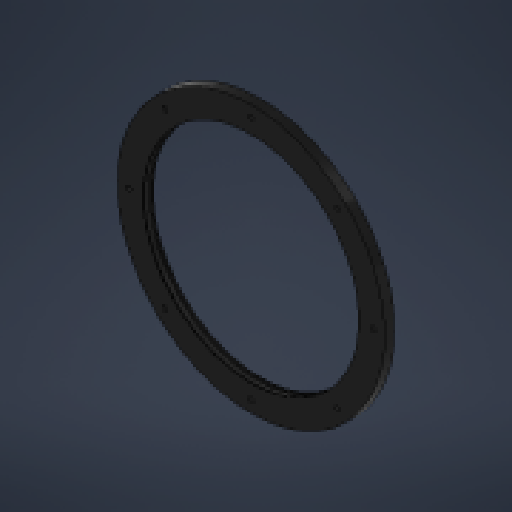
# Autodesk Inventor part: 3DPRINT,TURRET,BEARING,OUTER
Saved by Autodesk Inventor 2026 (Build 300175000, 175)
## iProperties
Created: 2026-02-09
Part Number: 3DPRINT,TURRET,BEARING,OUTER
Material: Nylon 6/6
Document SubType Name: Modeling
Designer: littl
Density: 1.13 g/cm^3
Appearance: Smooth - Black
Mass: 195.023 g
Surface Area: 545.104 cm^2
Volume: 172.587 cm^3
Author: littl
Autodesk Inventor part; units mm, degrees
ref_plane "YZ Plane" through (0, 0, 0) normal (1, 0, 0) x (0, 1, 0)
ref_plane "XZ Plane" through (0, 0, 0) normal (0, 1, 0) x (-1, 0, 0)
ref_plane "XY Plane" through (0, 0, 0) normal (0, 0, 1) x (1, 0, 0)
sketch "Sketch1" plane through (0, 0, 0) normal (1, 0, 0) x (0, 1, 0)
  arc A0 (-107.5189, 2.6268) -> (-107.5189, -2.6268) centre (-105.3147, 0) ccw
  line L0 (-105.5687, 3.175) -> (-105.5687, -3.175) construction
  line L1 (-107.5189, 2.6268) -> (-107.5189, 4.635) construction
  line L2 (-106.3625, 5.1846) -> (-106.3625, 3.5971)
  line L3 (-107.5189, 2.6268) -> (-106.3625, 3.5971)
  line L4 (-107.5189, -2.6268) -> (-106.3625, -3.5971)
  line L5 (-131.7625, 5.1846) -> (-131.7625, -5.1846)
  line L6 (-131.7625, 5.1846) -> (-106.3625, 5.1846)
  line L7 (-131.7625, -5.1846) -> (-106.3625, -5.1846)
  line L8 (-106.3625, -5.1846) -> (-106.3625, -3.5971)
  circle A1 centre (-105.5687, 0) radius 3.175 construction
  line L9 (-35.1032, 0) -> (87.3968, 0) construction
  line L10 (-104.775, 5.1846) -> (-104.775, 3.5971) construction
  line L11 (-104.775, -5.1846) -> (-104.775, -3.5971) construction
  line L12 (-103.6186, 2.6268) -> (-104.775, 3.5971) construction
  line L13 (-103.6186, -2.6268) -> (-104.775, -3.5971) construction
  arc A2 (-103.6186, -2.6268) -> (-103.6186, 2.6268) centre (-105.8227, 0) ccw construction
  line L14 (-79.375, 5.1846) -> (-79.375, -5.1846) construction
  line L15 (0, -7.2584) -> (0, 7.2584) construction
  line L16 (-79.375, -5.1846) -> (-104.775, -5.1846) construction
  line L17 (-79.375, 5.1846) -> (-104.775, 5.1846) construction
  line L18 (-104.775, 5.1846) -> (-104.775, 8.3596) construction
  line L19 (-104.775, 8.3596) -> (-79.375, 8.3596) construction
  line L20 (-79.375, 8.3596) -> (-79.375, 5.1846) construction
  line L21 (-90.4875, 22.7342) -> (-90.4875, 8.3596) construction
  point P0 (0, 0)
  point P1 (0, 0)
  point P2 (-108.7437, 0)
  point P3 (-131.7625, 0)
  point P4 (-19.1031, 0)
  point P5 (0, 7.2584)
  point P6 (0, 0)
  point P7 (-119.9381, 21.0485)
  dimension "d0" = 6.35
  dimension "d1" = 3.429
  dimension "d2" = 50
  dimension "d3" = 1.5875
  dimension "d4" = 1.5875
  dimension "d5" = 158.75
  dimension "d6" = 3.175
  dimension "d7" = 25.4
  dimension "d8" = 25.4
  dimension "d9" = 180.975
  constraints: 42 end point, 8 point on circle, 8 symmetric about line, 5 perpendicular, 5 vertical, 4 point on line, 3 centre point, 3 midpoint, 2 collinear, 2 horizontal alignment, 2 parallel, 2 tangent, 2 vertical alignment, 1 coincident, 1 horizontal, 6 other
  measures "d0" diameter of A1
  measures "d1" radius of A0
  measures "d2" angle of L3 L1
  measures "d3" distance of L7.end L4.end
  measures "d4" distance between parallel lines of L10 L2
  measures "d6" distance of L17.end L18.end
  measures "d7" distance of L18.end L19.end
  measures "d8" distance of L5.start L2.start
revolve "Revolution1" add sketch "Sketch1" angle 360 about axis through (0, 0, -7.2584) along (0, 0, 1)
sketch "Sketch2" plane through (0, 0, 5.1846) normal (0, 0, 1) x (1, 0, 0)
  point P0 (0, 0)
  point P1 (-120.65, 0)
  point P2 (-85.3124, -85.3124)
  point P3 (0, -120.65)
  point P4 (85.3124, -85.3124)
  point P5 (120.65, 0)
  point P6 (85.3124, 85.3124)
  point P7 (0, 120.65)
  point P8 (-85.3124, 85.3124)
  dimension "d11" = 120.65
  dimension "d14" = 360
  constraints: 1 horizontal alignment, 9 other
  measures "d11" distance of point (0, 0) point (-120.65, 0)
hole "Hole1" at (-120.65, 0, 5.1846) at (-85.3124, -85.3124, 5.1846) at (0, -120.65, 5.1846) at (85.3124, -85.3124, 5.1846) at (120.65, 0, 5.1846) at (85.3124, 85.3124, 5.1846) at (0, 120.65, 5.1846) at (-85.3124, 85.3124, 5.1846) direction (0, 0, -1) diameter 4.9784 end through all clearance for "Flat Head Machine Screw (82)" size "#10" standard "Ansi Unified Screw Threads"
thicken "Thicken1" operation cut thickness 0.7937 both sides no extend neighbours no toward (0, 0, -1) faces at (-13.7218, 118.4136, 5.1846)
equation "\"d8\" = d7"
body "Solid1"
